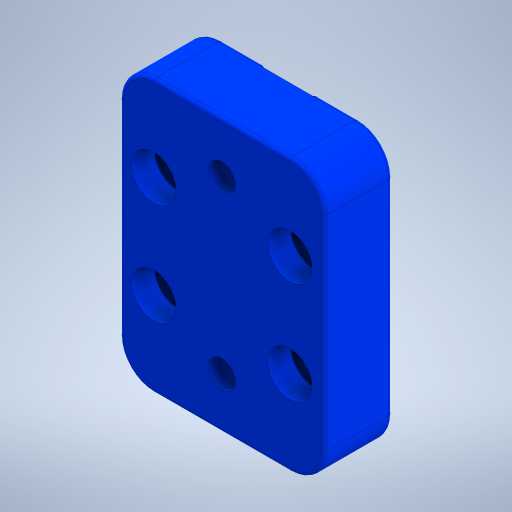
# Autodesk Inventor part: AdapterLinearGuideShort
Saved by Autodesk Inventor 2024 (Build 280153000, 153)
## iProperties
Created: 2023-12-27
Part Number: AdapterLinearGuideShort
Material: Generisch
Document SubType Name: Modeling
Designer: denni
Density: 1 g/cm^3
Appearance: Vorgabe(2)
Author: denni
Autodesk Inventor part; units mm, degrees
ref_plane "YZ Plane" through (0, 0, 0) normal (1, 0, 0) x (0, 1, 0)
ref_plane "XZ Plane" through (0, 0, 0) normal (0, 1, 0) x (-1, 0, 0)
ref_plane "XY Plane" through (0, 0, 0) normal (0, 0, 1) x (1, 0, 0)
sketch "Skizze1" plane through (0, 0, 0) normal (0, 0, 1) x (1, 0, 0)
  line L0 (0, 0) -> (30, 0)
  line L1 (30, 0) -> (30, 40)
  line L2 (30, 40) -> (0, 40)
  line L3 (0, 40) -> (0, 0)
  dimension "d0" = 30
  dimension "d1" = 40
  constraints: 8 end point, 2 parallel, 1 horizontal, 1 perpendicular
  measures "d0" distance of L1.end L2.end
  measures "d1" distance of L2.end L0.start
extrude "Extrusion1" add sketch "Skizze1" along normal blind 10
sketch "Skizze2" plane through (0, 0, 10) normal (0, 0, 1) x (1, 0, 0)
  line L0 (5, 27.5) -> (25, 27.5) construction
  line L1 (25, 27.5) -> (25, 12.5) construction
  line L2 (25, 12.5) -> (5, 12.5) construction
  line L3 (5, 12.5) -> (5, 27.5) construction
  line L4 (30, 40) -> (0, 40) construction
  line L5 (15, 27.5) -> (15, 40) construction
  line L6 (15, 12.5) -> (15, 0) construction
  line L7 (0, 0) -> (30, 0) projected
  dimension "d5" = 15
  dimension "d8" = 20
  constraints: 12 end point, 4 coincident, 4 midpoint, 2 parallel, 2 perpendicular, 1 collinear, 1 horizontal
  measures "d5" distance of L2.end L0.start
  measures "d8" distance of L0.start L0.end
hole "Bohrung1" at (5, 27.5, 10) at (25, 27.5, 10) at (25, 12.5, 10) at (5, 12.5, 10) direction (0, 0, -1) diameter 3.4 end through all counterbore diameter 6.5 counterbore depth 3.4 clearance for "Inbusschraube ISO 4762" size "M3" standard "ISO"
sketch "Skizze3" plane through (0, 0, 0) normal (0, 0, -1) x (-1, 0, 0)
  line L0 (-18.5, 40) -> (-11.5, 40)
  line L1 (-11.5, 40) -> (-11.5, 15)
  line L2 (-11.5, 15) -> (-18.5, 15)
  line L3 (-18.5, 15) -> (-18.5, 40)
  line L4 (-30, 40) -> (0, 40) projected
  point P0 (0, 0)
  point P1 (-15, 40)
  dimension "d19" = 7
  dimension "d20" = 25
  constraints: 8 end point, 2 midpoint, 2 parallel, 1 horizontal, 1 perpendicular
  measures "d19" distance of L1.end L2.end
  measures "d20" distance of L2.end L0.start
extrude "Extrusion2" cut sketch "Skizze3" against normal blind 0.5
fillet "Rundung3" radius 0.5 4 edges at (18.5, 40, 0.25) (11.5, 40, 0.25) (18.5, 15, 0.25) (11.5, 15, 0.25)
fillet "Rundung1" radius 5 4 edges at (0, 40, 5) (30, 40, 5) (0, 0, 5) (30, 0, 5)
fillet "Rundung2" radius 0.5 17 edges at (1.4645, 1.4645, 0) (15, 0, 0) (28.5355, 1.4645, 0) (30, 20, 0) (28.5355, 38.5355, 0) (8, 40, 0) (22, 40, 0) (1.4645, 38.5355, 0) (0, 20, 0) (1.4645, 38.5355, 10) (0, 20, 10) (1.4645, 1.4645, 10) (15, 0, 10) (28.5355, 1.4645, 10) (30, 20, 10) (28.5355, 38.5355, 10) (15, 40, 10)
sketch "Skizze4" plane through (0, 0, 10) normal (0, 0, 1) x (1, 0, 0)
  line L0 (19, 40) -> (11, 40) construction
  line L1 (15, 40) -> (15, 32.5) construction
  line L2 (15, 32.5) -> (15, 7.5) construction
  line L3 (15, 7.5) -> (15, 0) construction
  line L4 (25, 0) -> (5, 0) construction
  point P0 (0, 0)
  dimension "d24" = 25
  constraints: 6 end point, 2 coincident, 2 collinear, 2 midpoint, 1 perpendicular
  measures "d24" distance of L1.end L2.end
hole "Bohrung2" at (15, 32.5, 10) at (15, 7.5, 10) direction (0, 0, -1) diameter 4 end through all
